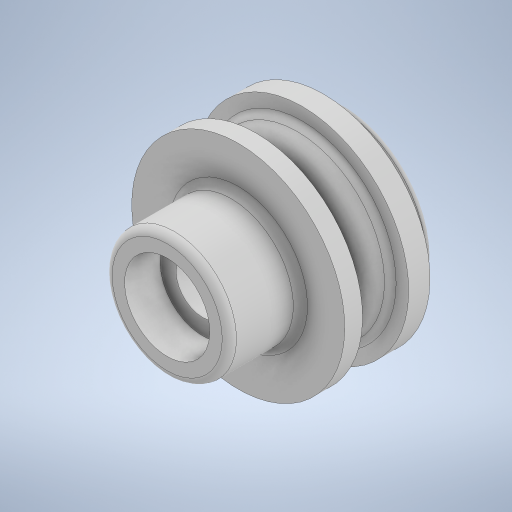
# Autodesk Inventor part: esercizio 02-27-2023
Saved by Autodesk Inventor 2023 (Build 270158000, 158)
## iProperties
Created: 2023-02-27
Part Number: esercizio 02-27-2023
Material: Generico
Document SubType Name: Modeling
Designer: Admin
Density: 1 g/cm^3
Appearance: Default
Author: Admin
Autodesk Inventor part; units mm, degrees
ref_plane "YZ Plane" through (0, 0, 0) normal (1, 0, 0) x (0, 1, 0)
ref_plane "XZ Plane" through (0, 0, 0) normal (0, 1, 0) x (-1, 0, 0)
ref_plane "XY Plane" through (0, 0, 0) normal (0, 0, 1) x (1, 0, 0)
sketch "Schizzo1" plane through (0, 0, 0) normal (1, 0, 0) x (0, 1, 0)
  line L0 (0, 0) -> (0, -15)
  line L1 (0, -15) -> (9, -15)
  line L2 (9, -15) -> (9, -7)
  line L3 (19, -32) -> (19, -22)
  line L4 (19, -22) -> (14.1471, -7)
  line L5 (19, -22) -> (34.7655, -22) construction
  line L6 (9, -7) -> (14.1471, -7)
  line L7 (19, -32) -> (25, -32)
  line L8 (25, -32) -> (25, -26)
  line L9 (25, -26) -> (30, -26)
  line L10 (30, -26) -> (30, -20)
  line L11 (30, -20) -> (25, -20)
  line L12 (25, -20) -> (20.7941, -7)
  line L13 (20.7941, -7) -> (30, -7)
  line L14 (30, -7) -> (30, -2)
  line L15 (30, -2) -> (17.5, -2)
  line L16 (17.5, -2) -> (17.5, 18)
  line L17 (17.5, 18) -> (12, 18)
  line L18 (12, 18) -> (12, 8)
  line L19 (12, 8) -> (7.5, 8)
  line L20 (7.5, 8) -> (7.5, 4)
  line L21 (7.5, 4) -> (12, 4)
  arc A0 (12.2479, 0) -> (12, 4) centre (12, 1.9923) ccw
  line L22 (12.2479, 0) -> (0, 0)
  point P0 (0, -7.5)
  point P1 (9.75, 8)
  point P2 (6.1239, 0)
  dimension "d3" = 15
  dimension "d7" = 10
  dimension "d10" = 18
  dimension "d11" = 38
  dimension "d12" = 50
  dimension "d13" = 60
  dimension "d14" = 25
  dimension "d15" = 6
  dimension "d16" = 6
  dimension "d17" = 25
  dimension "d18" = 50
  dimension "d19" = 20
  dimension "d20" = 10
  dimension "d23" = 15
  dimension "d24" = 24
  dimension "d25" = 35
  dimension "d26" = 60
  dimension "d27" = 4
  dimension "d28" = 18
  dimension "d29" = 12
  constraints: 46 end point, 11 perpendicular, 3 horizontal, 3 midpoint, 2 point on circle, 2 point on line, 1 centre point, 1 equal length, 1 parallel, 1 tangent, 1 vertical
  measures "d3" distance of L0.start L0.end
  measures "d7" distance of L3.start L3.end
  measures "d10" diameter of L2 L0
  measures "d11" diameter of L3 L0
  measures "d12" diameter of L8 L0
  measures "d13" diameter of L10 point (0, -7.5)
  measures "d14" distance between parallel lines of L7 L6
  measures "d15" distance of L7.end L8.end
  measures "d16" distance of L9.end L10.end
  measures "d17" distance between parallel lines of L7 L13
  measures "d18" distance between parallel lines of L7 L17
  measures "d19" distance between parallel lines of L17 L15
  measures "d20" distance from line of point (9.75, 8) L17
  measures "d23" diameter of L20 L0
  measures "d24" diameter of L18 L0
  measures "d25" diameter of L16 L0
  measures "d26" diameter of L14 L0
  measures "d27" distance between parallel lines of L22 L21
  measures "d28" distance from line of point (6.124, 0) L17
  measures "d29" distance between parallel lines of L7 L11
revolve "Rivoluzione1" add sketch "Schizzo1" angle 360 about axis through (0, 0, 0) along (0, 0, -1)
fillet "Raccordo1" radius 2 6 edges at (0, -25, -20) (0, -25, -32) (0, -25, -26) (0, -20.7941, -7) (0, -17.5, -2) (0, -17.5, 18)
